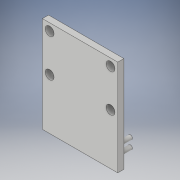
# Autodesk Inventor part: AS5047D
Saved by Autodesk Inventor 2019.1 (Build 231200000, 200)
## iProperties
Created: 2018-11-04
Part Number: AS5047D
Material: Generisch
Document SubType Name: Modeling
Designer: JochenAlt
Density: 1 g/cm^3
Appearance: Vorgabe
Author: JochenAlt
Autodesk Inventor part; units mm, degrees
ref_plane "YZ Plane" through (0, 0, 0) normal (1, 0, 0) x (0, 1, 0)
ref_plane "XZ Plane" through (0, 0, 0) normal (0, 1, 0) x (-1, 0, 0)
ref_plane "XY Plane" through (0, 0, 0) normal (0, 0, 1) x (1, 0, 0)
sketch "Skizze1" plane through (0, 0, 0) normal (0, 0, 1) x (1, 0, 0)
  line L0 (-11, 14) -> (11, 14)
  line L1 (11, 14) -> (11, -14)
  line L2 (11, -14) -> (-11, -14)
  line L3 (-11, -14) -> (-11, 14)
  line L4 (0, 19.6) -> (0, -19.6) construction
  line L5 (-15.4, 0) -> (15.4, 0) construction
  line L6 (-8.89, 0.89) -> (8.89, 0.89) construction
  line L7 (8.89, 0.89) -> (8.89, 11.89) construction
  line L8 (8.89, 11.89) -> (-8.89, 11.89) construction
  line L9 (-8.89, 11.89) -> (-8.89, 0.89) construction
  circle A0 centre (-8.89, 0.89) radius 1.3
  circle A1 centre (8.89, 0.89) radius 1.3
  circle A2 centre (8.89, 11.89) radius 1.3
  circle A3 centre (-8.89, 11.89) radius 1.3
  line L10 (-11, 14) -> (-8.89, 11.89) construction
  line L11 (-8.89, -11.46) -> (8.89, -11.46) construction
  line L12 (8.89, -11.46) -> (8.89, -8.92) construction
  line L13 (8.89, -8.92) -> (-8.89, -8.92) construction
  line L14 (-8.89, -8.92) -> (-8.89, -11.46) construction
  circle A4 centre (-8.89, -11.46) radius 0.6
  circle A5 centre (-6.35, -11.46) radius 0.6
  circle A6 centre (-3.81, -11.46) radius 0.6
  circle A7 centre (-1.27, -11.46) radius 0.6
  circle A8 centre (1.27, -11.46) radius 0.6
  circle A9 centre (3.81, -11.46) radius 0.6
  circle A10 centre (6.35, -11.46) radius 0.6
  circle A11 centre (8.89, -11.46) radius 0.6
  circle A12 centre (-8.89, -8.92) radius 0.6
  circle A13 centre (-6.35, -8.92) radius 0.6
  circle A14 centre (-3.81, -8.92) radius 0.6
  circle A15 centre (-1.27, -8.92) radius 0.6
  circle A16 centre (1.27, -8.92) radius 0.6
  circle A17 centre (3.81, -8.92) radius 0.6
  circle A18 centre (6.35, -8.92) radius 0.6
  circle A19 centre (8.89, -8.92) radius 0.6
  line L15 (-2, 4.64) -> (2, 4.64)
  line L16 (2, 4.64) -> (2, 8.14)
  line L17 (2, 8.14) -> (-2, 8.14)
  line L18 (-2, 8.14) -> (-2, 4.64)
  line L19 (-8.89, 0.89) -> (8.89, 11.89) construction
  line L20 (-8.89, 11.89) -> (8.89, 0.89) construction
  line L21 (-8.89, 6.39) -> (8.89, 6.39) construction
  point P0 (0, 0)
  point P1 (0, 6.39)
  dimension "d0" = 22
  dimension "d1" = 28
  dimension "d2" = 11
  dimension "d3" = 17.78
  dimension "d4" = 2.6
  dimension "d5" = 135
  dimension "d6" = 2.54
  dimension "d9" = 2.54
  dimension "d12" = 2.54
  dimension "d15" = 4
  dimension "d16" = 3.5
  dimension "d17" = 2.54
  dimension "d18" = 1.2
  constraints: 40 end point, 20 centre point, 8 parallel, 5 coincident, 5 horizontal, 4 midpoint, 4 perpendicular, 3 equal radius, 1 point on line, 1 vertical, 35 other
  measures "d0" distance of L1.end L2.end
  measures "d1" distance of L0.end L1.end
  measures "d2" distance of L6.end L7.end
  measures "d3" distance of L6.start L6.end
  measures "d4" diameter of A0
  measures "d5" angle of L3 L10
  measures "d6" distance between parallel lines of L13 L11
  measures "d9" distance of A4.centre A5.centre
  measures "d12" distance of A4.centre A12.centre
  measures "d15" distance of L16.end L17.end
  measures "d16" distance of L15.end L16.end
  measures "d17" distance from line of L2 L11.start
  measures "d18" diameter of A4
extrude "Extrusion1" add sketch "Skizze1" along normal blind 1.8 contours L0 L1 L2 L3 | A4 | A5 | A6 | A7 | A8 | A9 | A10 | A11 | A12 | A13 | A14 | A15 | A16 | A17 | A18 | A19 | L18 L17 L16 L15
extrude "Extrusion2" add sketch "Skizze1" against normal blind 4 from surface at 0 contours A4 | A5 | A6 | A7 | A8 | A9 | A10 | A11 | A12 | A13 | A14 | A15 | A16 | A17 | A18 | A19
extrude "Extrusion3" add sketch "Skizze1" against normal blind 1 from surface at 0 contours L18 L17 L16 L15
